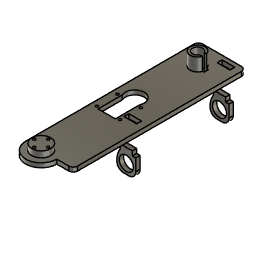
_Arm Limb 2 Dynamixel.92e19cb4-8085-4935-b305-b72b073291ea (Autodesk Fusion 360 design; units mm, degrees)
Autodesk Fusion 360 part; units mm, degrees
note: some values were not read from the file. Chosen so that the rebuilt part matches the saved one: which bodies a step acts on; which face or edge a step refers to. Set by a fixed rule: which sketch regions a step uses.
sketch "Sketch1" plane through (0, 0, 0) normal (0, 0, 1) x (1, 0, 0)
  circle A0 centre (25, 25) radius 1.5
  circle A1 centre (41, 25) radius 1.5
  circle A2 centre (33, 17) radius 1.5
  circle A3 centre (33, 33) radius 1.5
  circle A4 centre (33, 25) radius 18
  line L0 (15, 25) -> (51, 25)
  line L1 (51, 25) -> (51, 175)
  line L2 (51, 175) -> (15, 175)
  line L3 (15, 175) -> (15, 25)
  dimension "d1" = 3
  dimension "d2" = 3
  dimension "d3" = 3
  dimension "d4" = 3
  dimension "d5" = 36
  dimension "d6" = 150
  constraint horizontal L0
  constraint vertical L1
  constraint horizontal L2
  constraint vertical L3
  constraint coincident A4 L0.start
  measures "d1" diameter of A0
  measures "d2" diameter of A1
  measures "d3" diameter of A2
  measures "d4" diameter of A3
  measures "d5" distance of L0.start L0.end
  measures "d6" distance of L0.start L2.end
extrude "Extrude1" add sketch "Sketch1" along normal blind 5 contours A0 A1 A4 L0 | A0 A1 A4 L0 | A4 L1 L2 L3 makes body 1
sketch "Sketch4" plane through (0, 0, 0) normal (0, 0, 1) x (1, 0, 0)
  line L0 (50, 25) -> (70, 25)
  line L1 (70, 25) -> (70, 175)
  line L2 (70, 175) -> (50, 175)
  line L3 (50, 175) -> (50, 25)
  constraint horizontal L0
  constraint vertical L1
  constraint horizontal L2
  constraint vertical L3
extrude "Extrude3" add sketch "Sketch4" along normal blind 5 bodies 1
sketch "Sketch5" plane through (0, 0, 0) normal (0, 0, -1) x (1, 0, 0)
  line L0 (15, -175) -> (70, -175)
  line L1 (70, -175) -> (70, -25)
  line L2 (70, -25) -> (51, -25)
  arc A0 (51, -25) -> (15, -25) centre (33, -25) ccw
  line L3 (15, -25) -> (15, -175)
  circle A1 centre (33, -17) radius 1.5
  circle A2 centre (41, -25) radius 1.5
  circle A3 centre (25, -25) radius 1.5
  circle A4 centre (33, -33) radius 1.5
sketch "Sketch6" plane through (0, 0, 0) normal (0, 0, -1) x (1, 0, 0)
  line L0 (65.5, -170) -> (43.5, -170)
  line L1 (43.5, -170) -> (43.5, -165)
  line L2 (43.5, -165) -> (65.5, -165)
  line L3 (65.5, -165) -> (65.5, -170)
  line L4 (65.5, -62) -> (43.5, -62)
  line L5 (43.5, -62) -> (43.5, -57)
  line L6 (43.5, -57) -> (65.5, -57)
  line L7 (65.5, -57) -> (65.5, -62)
  dimension "d22" = 22
  dimension "d23" = 5
  dimension "d24" = 22
  dimension "d25" = 5
  constraint horizontal L0
  constraint vertical L1
  constraint horizontal L2
  constraint vertical L3
  constraint horizontal L4
  constraint vertical L5
  constraint horizontal L6
  constraint vertical L7
  measures "d22" distance of L0.start L0.end
  measures "d23" distance of L0.start L2.end
  measures "d24" distance of L4.start L4.end
  measures "d25" distance of L4.start L6.end
extrude "Extrude4" add sketch "Sketch6" along normal blind 22 bodies 1
sketch "Sketch7" plane through (0, 170, 0) normal (0, 1, 0) x (-1, 0, 0)
  line L0 (-43.5, 0) -> (-65.5, 0)
  line L1 (-65.5, 0) -> (-65.5, -22)
  line L2 (-65.5, -22) -> (-43.5, -22)
  line L3 (-43.5, -22) -> (-43.5, 0)
  circle A0 centre (-54.5, -11) radius 8.15
  dimension "d28" = 16.3
  measures "d28" diameter of A0
extrude "Extrude5" cut sketch "Sketch7" against normal blind 115 contours A0 bodies 1
fillet "Fillet1" radius 8 4 edges at (65.5, 167.5, -22) (43.5, 167.5, -22) (65.5, 59.5, -22) (43.5, 59.5, -22) on bodies 1
fillet "Fillet2" radius 5 3 edges at (70, 175, 2.5) (15, 175, 2.5) (70, 25, 2.5) on bodies 1
sketch "Sketch8" plane through (0, 0, 5) normal (0, 0, 1) x (-1, 0, 0)
  circle A0 centre (-33, -17) radius 1.5
  circle A1 centre (-41, -25) radius 1.5
  circle A2 centre (-25, -25) radius 1.5
  circle A3 centre (-33, -33) radius 1.5
  arc A4 (-65, -25) -> (-70, -30) centre (-65, -30) ccw
  line L0 (-70, -30) -> (-70, -170)
  arc A5 (-70, -170) -> (-65, -175) centre (-65, -170) ccw
  line L1 (-65, -175) -> (-20, -175)
  arc A6 (-20, -175) -> (-15, -170) centre (-20, -170) ccw
  line L2 (-15, -170) -> (-15, -25)
  arc A7 (-15, -25) -> (-51, -25) centre (-33, -25) ccw
  line L3 (-51, -25) -> (-65, -25)
  circle A8 centre (-39, -150) radius 5.8
  line L4 (-49.0301, -147.5429) -> (-43.0301, -147.5429)
  line L5 (-43.0301, -147.5429) -> (-43.0301, -152.5429)
  line L6 (-43.0301, -152.5429) -> (-49.0301, -152.5429)
  line L7 (-49.0301, -152.5429) -> (-49.0301, -147.5429)
  dimension "d35" = 11.6
  dimension "d42" = 6
  dimension "d43" = 5
  constraint horizontal L4
  constraint vertical L5
  constraint horizontal L6
  constraint vertical L7
  measures "d35" diameter of A8
  measures "d42" distance of L4.start L4.end
  measures "d43" distance of L4.start L6.end
extrude "Extrude6" cut sketch "Sketch8" against normal blind 5 contours A8 L4 L5 L6 | A8 L4 L5 L6 | A8 L4 L6 L7 bodies 1
sketch "Sketch9" plane through (0, 0, 5) normal (0, 0, 1) x (-1, 0, 0)
  arc A0 (-44.2129, -152.5429) -> (-44.2538, -147.5429) centre (-39, -150) ccw
  circle A1 centre (-33, -17) radius 1.5
  circle A2 centre (-41, -25) radius 1.5
  circle A3 centre (-25, -25) radius 1.5
  circle A4 centre (-33, -33) radius 1.5
  arc A5 (-65, -25) -> (-70, -30) centre (-65, -30) ccw
  line L0 (-70, -30) -> (-70, -170)
  arc A6 (-70, -170) -> (-65, -175) centre (-65, -170) ccw
  line L1 (-65, -175) -> (-20, -175)
  arc A7 (-20, -175) -> (-15, -170) centre (-20, -170) ccw
  line L2 (-15, -170) -> (-15, -25)
  arc A8 (-15, -25) -> (-51, -25) centre (-33, -25) ccw
  line L3 (-51, -25) -> (-65, -25)
  circle A9 centre (-39, -150) radius 8.6023
  line L4 (-49.0301, -147.5429) -> (-44.2538, -147.5429)
  line L5 (-44.2129, -152.5429) -> (-49.0301, -152.5429)
  line L6 (-49.0301, -152.5429) -> (-49.0301, -147.5429)
  constraint concentric A0 A9
extrude "Extrude7" add sketch "Sketch9" along normal blind 15 contours A0 A9 L4 L5 picked at (-31.3831, -150.7001) bodies 1
sketch "Sketch10" plane through (0, 0, 0) normal (0, 0, -1) x (1, 0, 0)
  line L0 (47.5, -170) -> (61.5, -170)
  line L1 (61.5, -170) -> (61.5, -165)
  line L2 (61.5, -165) -> (47.5, -165)
  line L3 (47.5, -165) -> (47.5, -170)
  line L4 (47.2, -170.3) -> (61.8, -170.3)
  line L5 (61.8, -170.3) -> (61.8, -164.7)
  line L6 (61.8, -164.7) -> (47.2, -164.7)
  line L7 (47.2, -164.7) -> (47.2, -170.3)
  line L8 (47.5, -62) -> (61.5, -62)
  line L9 (61.5, -62) -> (61.5, -57)
  line L10 (61.5, -57) -> (47.5, -57)
  line L11 (47.5, -57) -> (47.5, -62)
  line L12 (47.2, -62.3) -> (61.8, -62.3)
  line L13 (61.8, -62.3) -> (61.8, -56.7)
  line L14 (61.8, -56.7) -> (47.2, -56.7)
  line L15 (47.2, -56.7) -> (47.2, -62.3)
  dimension "d66" = 14.6
  dimension "d67" = 5.6
  constraint horizontal L0
  constraint vertical L1
  constraint horizontal L2
  constraint horizontal L4
  constraint vertical L5
  constraint horizontal L6
  constraint vertical L7
  constraint horizontal L8
  constraint vertical L9
  constraint horizontal L10
  constraint horizontal L12
  constraint vertical L13
  constraint horizontal L14
  constraint vertical L15
  measures "d66" distance of L5 L7
  measures "d67" distance of L4 L6
extrude "Extrude8" cut sketch "Sketch10" against normal blind 5 bodies 1
split "Split1" by plane through (0, 0, 0) normal (0, 0, 1) bodies 1 makes body 2 at (30.9124, 77.8968, 0) makes body 3 at (52.1667, 170, 1.6667) makes body 4 at (46.3905, 60.3333, -11.8115) makes body 5 at (52.1667, 60.3333, 5)
sketch "Sketch11" plane through (0, 0, 5) normal (0, 0, 1) x (-1, 0, 0)
  arc A0 (-45.7179, -152.5429) -> (-45.7439, -147.5429) centre (-37.5, -150) ccw
  line L0 (-45.7179, -152.5429) -> (-47.5301, -152.5429)
  line L1 (-47.5301, -152.5429) -> (-47.5301, -147.5429)
  line L2 (-47.5301, -147.5429) -> (-45.7439, -147.5429)
  circle A1 centre (-33, -17) radius 1.5
  circle A2 centre (-41, -25) radius 1.5
  circle A3 centre (-25, -25) radius 1.5
  circle A4 centre (-33, -33) radius 1.5
  arc A5 (-65, -25) -> (-70, -30) centre (-65, -30) ccw
  line L3 (-70, -30) -> (-70, -170)
  arc A6 (-70, -170) -> (-65, -175) centre (-65, -170) ccw
  line L4 (-65, -175) -> (-20, -175)
  arc A7 (-20, -175) -> (-15, -170) centre (-20, -170) ccw
  line L5 (-15, -170) -> (-15, -25)
  arc A8 (-15, -25) -> (-51, -25) centre (-33, -25) ccw
  line L6 (-51, -25) -> (-65, -25)
  circle A9 centre (-48, -75.3257) radius 1.5
  circle A10 centre (-21, -75.3257) radius 1.5
  circle A11 centre (-21, -51.3257) radius 1.5
  circle A12 centre (-48, -51.3257) radius 1.5
  line L7 (-47.2, -170.3) -> (-61.8, -170.3)
  line L8 (-61.8, -170.3) -> (-61.8, -164.7)
  line L9 (-61.8, -164.7) -> (-47.2, -164.7)
  line L10 (-47.2, -164.7) -> (-47.2, -170.3)
  line L11 (-47.2, -62.3) -> (-61.8, -62.3)
  line L12 (-61.8, -62.3) -> (-61.8, -56.7)
  line L13 (-61.8, -56.7) -> (-47.2, -56.7)
  line L14 (-47.2, -56.7) -> (-47.2, -62.3)
  circle A13 centre (-34.5, -81.8257) radius 11
  line L15 (-24.5, -49.3257) -> (-24.5, -77.2431)
  line L16 (-44.5, -49.3257) -> (-44.5, -77.2431)
  line L17 (-44.5, -49.3257) -> (-24.5, -49.3257)
  line L18 (-15, -175) -> (-15, -25)
  line L19 (-47.2, -170.3) -> (-61.8, -170.3)
  line L20 (-61.8, -170.3) -> (-61.8, -164.7)
  line L21 (-61.8, -164.7) -> (-47.2, -164.7)
  line L22 (-47.2, -164.7) -> (-47.2, -170.3)
  line L23 (-47.2, -62.3) -> (-61.8, -62.3)
  line L24 (-61.8, -62.3) -> (-61.8, -56.7)
  line L25 (-61.8, -56.7) -> (-47.2, -56.7)
  line L26 (-47.2, -56.7) -> (-47.2, -62.3)
  arc A14 (-47.2179, -152.5429) -> (-47.2439, -147.5429) centre (-39, -150) ccw
  line L27 (-47.2179, -152.5429) -> (-49.0301, -152.5429)
  line L28 (-49.0301, -152.5429) -> (-49.0301, -147.5429)
  line L29 (-49.0301, -147.5429) -> (-47.2439, -147.5429)
  circle A15 centre (-33, -17) radius 1.5
  circle A16 centre (-41, -25) radius 1.5
  circle A17 centre (-25, -25) radius 1.5
  circle A18 centre (-33, -33) radius 1.5
  arc A19 (-65, -25) -> (-70, -30) centre (-65, -30) ccw
  line L30 (-70, -30) -> (-70, -170)
  arc A20 (-70, -170) -> (-65, -175) centre (-65, -170) ccw
  line L31 (-65, -175) -> (-20, -175)
  arc A21 (-20, -175) -> (-15, -170) centre (-20, -170) ccw
  line L32 (-15, -170) -> (-15, -25)
  arc A22 (-15, -25) -> (-51, -25) centre (-33, -25) ccw
  line L33 (-51, -25) -> (-65, -25)
  dimension "d46" = 3
  dimension "d47" = 3
  dimension "d48" = 3
  dimension "d49" = 3
  dimension "d59" = 9.5
  dimension "d69" = 3.5
  dimension "d70" = 3.5
  dimension "d71" = 3.5
  dimension "d72" = 3.5
  constraint coincident A13 L15.end
  constraint vertical L15
  constraint coincident A13 L16.end
  constraint parallel L15 L16
  constraint perpendicular L16 L17
  measures "d46" diameter of A9
  measures "d47" diameter of A10
  measures "d48" diameter of A11
  measures "d49" diameter of A12
  measures "d59" distance of L5 L15
  measures "d69" distance of A10.centre L15
  measures "d70" distance of A9.centre L16
  measures "d71" distance of A12.centre L16
  measures "d72" distance of A11.centre L15
extrude "Extrude9" cut sketch "Sketch11" against normal blind 5 contours A9 | A10 | A11 | A12 | A13 | A13 L15 L16 L17 bodies 2
move_body "Move5" bodies 4 1 to x (1, 0, 0) y (0, 1, 0) z (0, 0, 1) at (0, 0, -25)
move_body "Move6" bodies 3 5 to x (1, 0, 0) y (0, 1, 0) z (0, 0, 1) at (0, 0, -25)
combine "Combine7" operation add target body 1 tool bodies 3
combine "Combine8" operation add target body 5 tool bodies 4
sketch "Sketch12" plane through (0, 0, 5) normal (0, 0, 1) x (-1, 0, 0)
  circle A0 centre (-48, -75.3257) radius 1.5
  circle A1 centre (-21, -75.3257) radius 1.5
  circle A2 centre (-48, -51.3257) radius 1.5
  circle A3 centre (-21, -51.3257) radius 1.5
  line L0 (-47.2, -170.3) -> (-61.8, -170.3)
  line L1 (-61.8, -170.3) -> (-61.8, -164.7)
  line L2 (-61.8, -164.7) -> (-47.2, -164.7)
  line L3 (-47.2, -164.7) -> (-47.2, -170.3)
  line L4 (-47.2, -62.3) -> (-61.8, -62.3)
  line L5 (-61.8, -62.3) -> (-61.8, -56.7)
  line L6 (-61.8, -56.7) -> (-47.2, -56.7)
  line L7 (-47.2, -56.7) -> (-47.2, -62.3)
  arc A4 (-47.2179, -152.5429) -> (-47.2439, -147.5429) centre (-39, -150) ccw
  line L8 (-47.2179, -152.5429) -> (-49.0301, -152.5429)
  line L9 (-49.0301, -152.5429) -> (-49.0301, -147.5429)
  line L10 (-49.0301, -147.5429) -> (-47.2439, -147.5429)
  circle A5 centre (-33, -17) radius 1.5
  circle A6 centre (-41, -25) radius 1.5
  circle A7 centre (-25, -25) radius 1.5
  circle A8 centre (-33, -33) radius 1.5
  arc A9 (-65, -25) -> (-70, -30) centre (-65, -30) ccw
  line L11 (-70, -30) -> (-70, -170)
  arc A10 (-70, -170) -> (-65, -175) centre (-65, -170) ccw
  line L12 (-65, -175) -> (-20, -175)
  arc A11 (-20, -175) -> (-15, -170) centre (-20, -170) ccw
  line L13 (-15, -170) -> (-15, -25)
  arc A12 (-15, -25) -> (-51, -25) centre (-33, -25) ccw
  line L14 (-51, -25) -> (-65, -25)
  circle A13 centre (-33, -25) radius 11
  line L15 (-44.5, -49.3257) -> (-24.5, -49.3257)
  line L16 (-24.5, -49.3257) -> (-24.5, -77.2431)
  line L17 (-44.5, -77.2431) -> (-44.5, -49.3257)
  arc A14 (-44.5, -77.2431) -> (-24.5, -77.2431) centre (-34.5, -81.8257) ccw
  dimension "d52" = 22
  constraint concentric A12 A13
  measures "d52" diameter of A13
extrude "Extrude10" add sketch "Sketch12" along normal blind 7 contours A13 bodies 2
move_body "Move7" bodies 2 to x (1, 0, 0) y (0, 1, 0) z (0, 0, 1) at (0, -45, 0)
split "Split2" by plane through (0, 0, 0) normal (0, 1, 0) bodies 2 makes body 6 at (60.2767, 81.6143, 0)
move_body "Move8" bodies 6 to x (1, 0, 0) y (0, 1, 0) z (0, 0, 1) at (0, 50, 0)
extrude "Extrude11" add 1 faces at (51.6667, 0, 1.6667) along direction (0, 1, 0) blind 50 on bodies 2 bodies 2 6
chamfer "Chamfer1" distance 4 angle 45 2 edges at (43.5, 59.5, -25) (43.5, 167.5, -25) on bodies 1 5
fillet "Fillet3" radius 25 2 edges at (43.5, 167.5, -29) (43.5, 59.5, -29) on bodies 1 5
equation "d59 = 8 mm + 1.5 mm"
